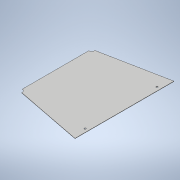
# Autodesk Inventor part: Firewalltrapezoid2
Saved by Autodesk Inventor 2021 (Build 250183000, 183)
## iProperties
Created: 2020-10-29
Part Number: Firewalltrapezoid2
Material: Generic
Document SubType Name: Modeling
Designer: mackeycj
Density: 1 g/cm^3
Appearance: Default
Author: mackeycj
Autodesk Inventor part; units mm, degrees
ref_plane "YZ Plane" through (0, 0, 0) normal (1, 0, 0) x (0, 1, 0)
ref_plane "XZ Plane" through (0, 0, 0) normal (0, 1, 0) x (-1, 0, 0)
ref_plane "XY Plane" through (0, 0, 0) normal (0, 0, 1) x (1, 0, 0)
sketch "Sketch1" plane through (0, 0, 0) normal (0, 1, 0) x (-1, 0, 0)
  line L0 (0, 0) -> (389.255, 0)
  line L1 (0, 0) -> (0, -279.4)
  line L2 (0, 0) -> (0, 279.4)
  line L3 (389.255, 0) -> (389.255, 203.2)
  line L4 (389.255, 0) -> (389.255, -203.2)
  line L5 (389.255, -203.2) -> (0, -279.4)
  line L6 (389.255, 203.2) -> (0, 279.4)
  line L7 (0, 279.4) -> (169.2753, 246.2629)
  line L8 (169.2753, 246.2629) -> (296.4024, 221.3767)
  circle A0 centre (389.255, 203.2) radius 15.875
  circle A1 centre (389.255, -203.2) radius 15.875
  line L9 (0, -279.4) -> (169.2753, -246.2629)
  line L10 (169.2753, -246.2629) -> (296.4024, -221.3767)
  point P0 (373.6757, -206.2498)
  point P1 (389.255, -187.325)
  point P2 (389.255, 187.325)
  point P3 (373.6757, 206.2498)
  dimension "d12" = 389.255
  dimension "d13" = 279.4
  dimension "d14" = 279.4
  dimension "d15" = 203.2
  dimension "d16" = 203.2
  dimension "d23" = 31.75
  dimension "d24" = 31.75
  dimension "d26" = 129.54
  constraints: 22 end point, 4 point on line, 4 vertical, 3 coincident, 2 centre point, 1 horizontal
  measures "d12" distance of L0.start L0.end
  measures "d13" distance of L0.start L1.end
  measures "d14" distance of L0.start L2.end
  measures "d15" distance of L0.end L3.end
  measures "d16" distance of L0.end L4.end
  measures "d23" diameter of A0
  measures "d24" diameter of A1
  measures "d26" distance of L9.end L10.end
extrude "Extrusion1" add sketch "Sketch1" along normal blind 1.524 contours L2 L6 A0 L3 L0 | L0 L4 A1 L5 L1
sketch "Sketch2" plane through (0, 0, 0) normal (0, 1, 0) x (-1, 0, 0)
  line L0 (0, 0) -> (0, 203.2)
  line L1 (0, 279.4) -> (0, -279.4) projected
  line L2 (0, 203.2) -> (19.05, 203.2)
  circle A0 centre (19.05, 203.2) radius 4.7625
  line L3 (0, 0) -> (0, -203.2)
  line L4 (0, -203.2) -> (19.05, -203.2)
  circle A1 centre (19.05, -203.2) radius 4.7625
  line L5 (389.255, -187.325) -> (389.255, 187.325) projected
  line L6 (389.255, 0) -> (389.255, 203.2)
  line L7 (389.255, 203.2) -> (370.205, 203.2)
  line L8 (389.255, 0) -> (389.255, -203.2)
  line L9 (389.255, -203.2) -> (370.205, -203.2)
  dimension "d29" = 203.2
  dimension "d30" = 19.05
  dimension "d31" = 9.525
  dimension "d32" = 203.2
  dimension "d33" = 19.05
  dimension "d34" = 9.525
  dimension "d35" = 203.2
  dimension "d36" = 19.05
  dimension "d37" = 203.2
  dimension "d38" = 19.05
  constraints: 16 end point, 4 perpendicular, 4 point on line, 2 centre point, 2 coincident, 1 midpoint
  measures "d29" distance of L0.start L0.end
  measures "d30" distance of L0.end L2.end
  measures "d31" diameter of A0
  measures "d32" distance of L0.start L3.end
  measures "d33" distance of L3.end L4.end
  measures "d34" diameter of A1
  measures "d35" distance of L6.start L6.end
  measures "d36" distance of L6.end L7.end
  measures "d37" distance of L6.start L8.end
  measures "d38" distance of L8.end L9.end
extrude "Extrusion2" cut sketch "Sketch2" along normal blind 25.4
body "Solid1"
